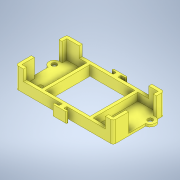
# Autodesk Inventor part: Battery-Holder-2x2
Saved by Autodesk Inventor 2022 (Build 260153000, 153)
## iProperties
Created: 2024-07-10
Part Number: Battery-Holder-2x2
Material: 一般
Document SubType Name: Modeling
Designer: yamashita1
Density: 1 g/cm^3
Appearance: 滑らか - 黄
Author: yamashita1
Autodesk Inventor part; units mm, degrees
ref_plane "YZ Plane" through (0, 0, 0) normal (1, 0, 0) x (0, 1, 0)
ref_plane "XZ Plane" through (0, 0, 0) normal (0, 1, 0) x (-1, 0, 0)
ref_plane "XY Plane" through (0, 0, 0) normal (0, 0, 1) x (1, 0, 0)
sketch "スケッチ1" plane through (0, 0, 0) normal (0, 0, 1) x (1, 0, 0)
  line L0 (-44.3295, 0) -> (44.3295, 0) construction
  line L1 (0, 23.7122) -> (0, -23.7122) construction
  line L2 (-26.6016, -16.95) -> (26.6016, -16.95) construction
  line L3 (-23, 17.7575) -> (-23, -30.8175) construction
  line L4 (23, -30.8175) -> (23, 17.7575) construction
  line L5 (-31, 17.7575) -> (-31, -30.8175) construction
  line L6 (31, -30.8175) -> (31, 17.7575) construction
  circle A0 centre (-31, 0) radius 1.6
  circle A1 centre (-23, -16.95) radius 1.6
  circle A2 centre (23, -16.95) radius 1.6
  circle A3 centre (31, 0) radius 1.6
  line L7 (-29.5, 6.55) -> (29.5, 6.55)
  line L8 (29.5, 6.55) -> (29.5, -22.45)
  line L9 (29.5, -22.45) -> (-29.5, -22.45)
  line L10 (-29.5, -22.45) -> (-29.5, 6.55)
  circle A4 centre (-23, -16.95) radius 3.5
  circle A5 centre (-31, 0) radius 3.5
  circle A6 centre (23, -16.95) radius 3.5
  circle A7 centre (31, 0) radius 3.5
  line L11 (-31.5, 8.55) -> (31.5, 8.55)
  line L12 (-31.5, 8.55) -> (-31.5, -24.45)
  line L13 (31.5, 8.55) -> (31.5, -24.45)
  line L14 (-31.5, -24.45) -> (31.5, -24.45)
  line L15 (-23, -20.45) -> (23, -20.45)
  line L16 (-26.5, -22.45) -> (-26.5, -24.45)
  line L17 (26.5, -24.45) -> (26.5, -22.45)
  line L18 (-31.5, -14.45) -> (-29.5, -14.45)
  line L19 (-31.5, 3.5) -> (-29.5, 3.5)
  line L20 (29.5, 3.5) -> (31.5, 3.5)
  line L21 (29.5, -14.45) -> (31.5, -14.45)
  line L22 (-21.5, 8.55) -> (-21.5, 6.55)
  line L23 (23.5, 8.55) -> (23.5, 6.55)
  line L24 (-16.5, 8.55) -> (-16.5, -24.45)
  line L25 (-14.5, -24.45) -> (-14.5, 8.55)
  line L26 (16.5, 8.55) -> (16.5, -24.45)
  line L27 (14.5, -24.45) -> (14.5, 8.55)
  line L28 (-40.1456, -7.95) -> (40.1456, -7.95) construction
  line L29 (-1.5, 8.55) -> (-1.5, 10.55)
  line L30 (-1.5, 10.55) -> (-4.5, 10.55)
  line L31 (-4.5, 10.55) -> (-4.5, 11.75)
  line L32 (-4.5, 11.75) -> (4.5, 11.75)
  line L33 (4.5, 11.75) -> (4.5, 10.55)
  line L34 (4.5, 10.55) -> (1.5, 10.55)
  line L35 (1.5, 10.55) -> (1.5, 8.55)
  line L36 (-1.5, -24.45) -> (-1.5, -26.45)
  line L37 (-1.5, -26.45) -> (-4.5, -26.45)
  line L38 (-4.5, -26.45) -> (-4.5, -27.65)
  line L39 (-4.5, -27.65) -> (4.5, -27.65)
  line L40 (4.5, -27.65) -> (4.5, -26.45)
  line L41 (4.5, -26.45) -> (1.5, -26.45)
  line L42 (1.5, -26.45) -> (1.5, -24.45)
  point P0 (0, 0)
  point P1 (0, 0)
  point P2 (0, -16.95)
  point P3 (0, -22.45)
  point P4 (-31.5, 3.4641)
  point P5 (-31.5, -3.4641)
  point P6 (-26.3541, -17.95)
  point P7 (26.3541, -17.95)
  point P8 (31.5, -3.4641)
  point P9 (31.5, 3.4641)
  point P10 (29.5, -3.1623)
  point P11 (25.8723, -14.95)
  point P12 (-19.6459, -17.95)
  point P13 (19.6459, -17.95)
  point P14 (20.1277, -14.95)
  point P15 (-20.1277, -14.95)
  point P16 (-25.8723, -14.95)
  point P17 (-29.5, -3.1623)
  point P18 (29.5, 3.1623)
  point P19 (-29.5, 3.1623)
  point P20 (0, -7.95)
  point P21 (16.5, -22.45)
  point P22 (14.5, -22.45)
  point P23 (-14.5, -22.45)
  point P24 (-16.5, -22.45)
  point P25 (16.5, 6.55)
  point P26 (14.5, 6.55)
  point P27 (-14.5, 6.55)
  point P28 (-16.5, 6.55)
  point P29 (14.5, -20.45)
  point P30 (-14.5, -20.45)
  dimension "MOUNT_W" = 16.95
  dimension "d1" = 23
  dimension "d2" = 31
  dimension "d3" = 3.2
  dimension "d4" = 59
  dimension "d5" = 29
  dimension "d8" = 7
  dimension "d9" = 2
  dimension "d10" = 2
  dimension "d11" = 2
  dimension "d12" = 2
  dimension "d18" = 8
  dimension "d19" = 8
  dimension "d20" = 8
  dimension "d24" = 2
  dimension "d25" = 2
  dimension "d26" = 2
  dimension "d27" = 13
  dimension "d28" = 13
  dimension "d33" = 3
  dimension "d34" = 9
  dimension "d35" = 2
  dimension "d36" = 1.2
  constraints: 82 end point, 32 point on line, 16 perpendicular, 16 vertical, 6 centre point, 6 horizontal, 5 coincident, 5 collinear, 5 midpoint, 3 equal radius, 2 parallel, 1 tangent, 41 other
  measures "MOUNT_W" distance between parallel lines of L2 L0
  measures "d1" distance between parallel lines of L3 L1
  measures "d2" distance from line of L5.end L1
  measures "d3" diameter of A0
  measures "d4" distance of L8.end L9.end
  measures "d5" distance of L7.end L8.end
  measures "d8" diameter of A5
  measures "d10" distance between parallel lines of L12 L10
  measures "d11" distance between parallel lines of L13 L8
  measures "d18" distance between parallel lines of L9 L18
  measures "d19" distance between parallel lines of L10 L22
  measures "d20" distance between parallel lines of L13 L23
  measures "d24" distance between parallel lines of L9 L15
  measures "d25" distance between parallel lines of L24 L25
  measures "d26" distance between parallel lines of L27 L26
  measures "d27" distance between parallel lines of L26 L8
  measures "d28" distance between parallel lines of L10 L24
  measures "d33" distance between parallel lines of L35 L29
  measures "d34" distance of L31.end L32.end
  measures "d35" distance of L29.start L29.end
  measures "d36" distance of L30.end L31.end
extrude "ベース" add sketch "スケッチ1" against normal blind 1.5 contours A0 L10 A5 | A0 L12 A5 L10 | L10 A5 L12 A0 | A0 L12 A5 | A5 L19 L10 | L10 L7 L24 L9 A5 | L10 L18 L12 A5 | L12 L19 A5 | L19 L12 L11 L22 L7 L10 | L10 L9 L16 L14 L12 L18 | L22 L11 L24 L7 | L9 L24 L14 L16 | L24 L11 L25 L7 | L7 L25 L15 L24 | L24 L15 L25 L9 | L9 L25 L14 L24 | L25 L11 L27 L7 | L7 L27 L15 L25 | L25 L15 L27 L9 | L9 L27 L14 L25 | L27 L11 L26 L7 | L7 L26 L15 L27 | L27 L15 L26 L9 | L9 L26 L14 L27 | L26 L11 L23 L7 | L7 L8 A7 L9 L26 | L9 L17 L14 L26 | L23 L11 L13 L20 L8 L7 | L9 L8 L21 L13 L14 L17 | L20 A7 L8 | L8 A7 L13 L21 | A7 L13 A3 L8 | L8 A3 A7 | L20 L13 A7 | L8 A3 L13 A7 | A7 L13 A3 | A4 | A6
extrude "囲い柱" add sketch "スケッチ1" along normal blind 12 contours L19 L12 L11 L22 L7 L10 | L10 L9 L16 L14 L12 L18 | L23 L11 L13 L20 L8 L7 | L9 L8 L21 L13 L14 L17
extrude "底上げ" add sketch "スケッチ1" along normal blind 5 contours L22 L11 L24 L7 | L9 L24 L14 L16 | L24 L11 L25 L7 | L7 L25 L15 L24 | L24 L15 L25 L9 | L9 L25 L14 L24 | L25 L11 L27 L7 | L9 L27 L14 L25 | L27 L11 L26 L7 | L7 L26 L15 L27 | L27 L15 L26 L9 | L9 L26 L14 L27 | L26 L11 L23 L7 | L9 L17 L14 L26
extrude "肉抜き" cut sketch "スケッチ1" against normal through all contours L7 L27 L15 L25 | L25 L15 L27 L9
extrude "輪ゴムタブ" add sketch "スケッチ1" along normal blind 5 and the other way blind 1.5 contours L29 L30 L31 L32 L33 L34 L35 L11 | L14 L42 L41 L40 L39 L38 L37 L36
fillet "フィレット1" radius 1.5 4 edges at (-31.5, 8.55, 5.25) (31.5, 8.55, 5.25) (-31.5, -24.45, 5.25) (31.5, -24.45, 5.25)
fillet "フィレット2" radius 0.5 15 edges at (-4.5, 11.75, 1.75) (-4.5, 10.55, 1.75) (4.5, 10.55, 1.75) (4.5, 11.75, 1.75) (1.5, 10.55, 1.75) (1.5, 8.55, 1.75) (-1.5, 10.55, 1.75) (-1.5, 8.55, 1.75) (-1.5, -26.45, 1.75) (-4.5, -26.45, 1.75) (-4.5, -27.65, 1.75) (4.5, -26.45, 1.75) (1.5, -24.45, 1.75) (4.5, -27.65, 1.75) (1.5, -26.45, 1.75)
equation "\"d5\" = BAT_W + CLEARANCE"
equation "\"d9\" = TAB_W"
equation "\"d10\" = d9"
equation "\"d11\" = d9"
equation "\"d12\" = d9"
equation "\"d18\" = d19"
equation "\"d20\" = d19"
equation "\"d26\" = d25"
equation "\"d28\" = d27"
equation "\"d22\" = TAB_H"
equation "\"BAT_L\" = 58"
equation "\"BAT_W\" = 28"
equation "\"CLEARANCE\" = 1"
equation "\"TAB_W\" = 2"
equation "\"TAB_H\" = 12"
